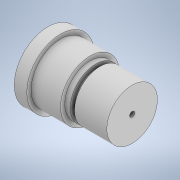
# Autodesk Inventor part: 1
Saved by Autodesk Inventor 2020 (Build 240168000, 168)
## iProperties
Created: 2022-04-06
Part Number: 1
Material: Типовые
Document SubType Name: Modeling
Designer: User
Density: 1 g/cm^3
Appearance: По умолчанию
Author: User
Autodesk Inventor part; units mm, degrees
ref_plane "YZ Plane" through (0, 0, 0) normal (1, 0, 0) x (0, 1, 0)
ref_plane "XZ Plane" through (0, 0, 0) normal (0, 1, 0) x (-1, 0, 0)
ref_plane "XY Plane" through (0, 0, 0) normal (0, 0, 1) x (1, 0, 0)
sketch "Эскиз1" plane through (0, 0, 0) normal (0, 0, 1) x (1, 0, 0)
  line L0 (0, 0) -> (100, 0)
  line L1 (100, 0) -> (100, 30)
  line L2 (100, 30) -> (50, 30)
  line L3 (50, 30) -> (50, 35)
  line L4 (50, 35) -> (15, 35)
  line L5 (15, 35) -> (15, 40)
  line L6 (15, 40) -> (0, 40)
  line L7 (0, 40) -> (0, 0)
  line L8 (56.6884, 30) -> (56.6884, 25)
  line L9 (56.6884, 25) -> (61.6884, 25)
  line L10 (61.6884, 25) -> (61.6884, 30)
  dimension "d0" = 100
  dimension "d1" = 30
  dimension "d2" = 50
  dimension "d3" = 5
  dimension "d4" = 35
  dimension "d5" = 5
  dimension "d7" = 5
  dimension "d8" = 5
  dimension "d9" = 11.6884
  constraints: 22 end point, 10 perpendicular, 2 point on line, 1 horizontal
  measures "d0" distance of L0.start L0.end
  measures "d1" distance of L0.end L1.end
  measures "d2" distance of L1.end L2.end
  measures "d3" distance of L2.end L3.end
  measures "d4" distance of L3.end L4.end
  measures "d5" distance of L4.end L5.end
  measures "d7" distance of L8.start L8.end
  measures "d8" distance of L8.end L9.end
  measures "d9" distance between parallel lines of L3 L10
revolve "Вращение1" add sketch "Эскиз1" angle 360 about axis through (0, 0, 0) along (1, 0, 0)
revolve "Вращение2" cut sketch "Эскиз1" angle 360 about axis through (0, 0, 0) along (-1, 0, 0) contours L10 L9 L8 L2
sketch "Эскиз2" plane through (0, 0, 0) normal (1, 0, 0) x (0, 1, 0)
  circle A0 centre (0, 0) radius 3
  dimension "d11" = 6
  constraints: 1 centre point, 1 coincident
  measures "d11" diameter of A0
extrude "Выдавливание1" cut sketch "Эскиз2" along normal up to surface (100 mm away)
